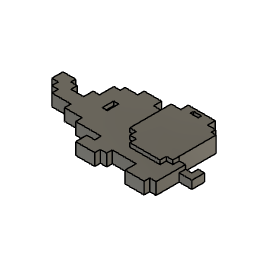
elephant pixel keychain v1 (Autodesk Fusion 360 design; units mm, degrees)
Autodesk Fusion 360 part; units mm, degrees
sketch "elephant sketch" plane through (0, 0, 0) normal (0, 0, 1) x (1, 0, 0)
  line L0 (5, 40) -> (5, 33)
  line L1 (5, 33) -> (9, 33)
  line L2 (9, 33) -> (9, 29)
  line L3 (9, 29) -> (13, 29)
  line L4 (13, 29) -> (13, 25)
  line L5 (13, 25) -> (25, 25)
  line L6 (25, 25) -> (25, 21)
  line L7 (25, 21) -> (36, 21)
  line L8 (36, 21) -> (36, 17)
  line L9 (36, 17) -> (52, 17)
  line L10 (52, 17) -> (52, 13)
  line L11 (52, 13) -> (47, 13)
  line L12 (47, 13) -> (47, 6)
  line L13 (47, 6) -> (59, 6)
  line L14 (59, 6) -> (59, 9.5)
  line L15 (59, 9.5) -> (63, 9.5)
  line L16 (63, 9.5) -> (63, 13)
  line L17 (63, 13) -> (78, 13)
  line L18 (78, 13) -> (78, 6)
  line L19 (78, 6) -> (90, 6)
  line L20 (90, 6) -> (90, 9.5)
  line L21 (90, 9.5) -> (94, 9.5)
  line L22 (94, 9.5) -> (94, 28)
  line L23 (94, 28) -> (90, 28)
  line L24 (90, 28) -> (90, 24)
  line L25 (90, 24) -> (86, 24)
  line L26 (86, 24) -> (86, 20)
  line L27 (86, 20) -> (67, 20)
  line L28 (67, 20) -> (67, 24)
  line L29 (67, 24) -> (63, 24)
  line L30 (63, 24) -> (63, 28)
  line L31 (63, 28) -> (59, 28)
  line L32 (59, 28) -> (59, 50)
  line L33 (59, 50) -> (52, 50)
  line L34 (52, 50) -> (52, 55)
  line L35 (52, 55) -> (41, 55)
  line L36 (41, 55) -> (41, 51)
  line L37 (41, 51) -> (33, 51)
  line L38 (33, 51) -> (33, 48)
  line L39 (33, 48) -> (29, 48)
  line L40 (29, 48) -> (29, 39)
  line L41 (29, 39) -> (25, 39)
  line L42 (25, 39) -> (25, 33)
  line L43 (25, 33) -> (17, 33)
  line L44 (17, 33) -> (17, 37)
  line L45 (17, 37) -> (13, 37)
  line L46 (13, 37) -> (13, 40)
  line L47 (13, 40) -> (5, 40)
  line L48 (94, 28) -> (98, 28)
  line L49 (98, 28) -> (98, 32)
  line L50 (98, 32) -> (102, 32)
  line L51 (102, 32) -> (102, 24)
  line L52 (102, 24) -> (94, 24)
  line L53 (59, 50) -> (59, 54)
  line L54 (59, 54) -> (65, 54)
  line L55 (65, 54) -> (65, 58.7382)
  line L56 (65, 58.7382) -> (81.9319, 58.7382)
  line L57 (81.9319, 58.7382) -> (81.9319, 54)
  line L58 (81.9319, 54) -> (87.0128, 54)
  line L59 (87.0128, 54) -> (87.0128, 51.2757)
  line L60 (87.0128, 51.2757) -> (90, 51.2757)
  line L61 (90, 51.2757) -> (90, 28)
  line L62 (36.8391, 40.0538) -> (36.8391, 32.8575)
  line L63 (36.8391, 32.8575) -> (40, 32.8575)
  line L64 (40, 32.8575) -> (40, 40.0538)
  line L65 (40, 40.0538) -> (36.8391, 40.0538)
  line L66 (71, 57) -> (75, 57)
  line L67 (75, 57) -> (75, 55)
  line L68 (75, 55) -> (70, 55)
  line L69 (70, 55) -> (70, 57)
  line L70 (70, 57) -> (71, 57)
  constraint vertical L0
  constraint perpendicular L0 L1
  constraint perpendicular L1 L2
  constraint perpendicular L0 L3
  constraint perpendicular L3 L4
  constraint perpendicular L0 L5
  constraint perpendicular L5 L6
  constraint perpendicular L6 L7
  constraint perpendicular L7 L8
  constraint perpendicular L8 L9
  constraint perpendicular L9 L10
  constraint perpendicular L10 L11
  constraint perpendicular L11 L12
  constraint perpendicular L12 L13
  constraint perpendicular L13 L14
  constraint perpendicular L14 L15
  constraint perpendicular L13 L16
  constraint perpendicular L16 L17
  constraint perpendicular L13 L18
  constraint perpendicular L18 L19
  constraint perpendicular L19 L20
  constraint perpendicular L20 L21
  constraint perpendicular L21 L22
  constraint perpendicular L22 L23
  constraint perpendicular L23 L24
  constraint perpendicular L22 L25
  constraint perpendicular L23 L26
  constraint perpendicular L22 L27
  constraint perpendicular L23 L28
  constraint perpendicular L28 L29
  constraint perpendicular L23 L30
  constraint perpendicular L30 L31
  constraint perpendicular L23 L32
  constraint perpendicular L30 L33
  constraint perpendicular L23 L34
  constraint perpendicular L34 L35
  constraint perpendicular L35 L36
  constraint perpendicular L34 L37
  constraint perpendicular L37 L38
  constraint perpendicular L38 L39
  constraint perpendicular L39 L40
  constraint perpendicular L38 L41
  constraint perpendicular L41 L42
  constraint perpendicular L42 L43
  constraint perpendicular L41 L44
  constraint perpendicular L44 L45
  constraint perpendicular L41 L46
  constraint perpendicular L0 L47
  constraint perpendicular L22 L48
  constraint perpendicular L23 L49
  constraint perpendicular L49 L50
  constraint perpendicular L50 L51
  constraint coincident L22 L52.end
  constraint perpendicular L22 L52
  constraint perpendicular L33 L53
  constraint perpendicular L32 L54
  constraint perpendicular L54 L55
  constraint perpendicular L55 L56
  constraint perpendicular L54 L57
  constraint perpendicular L57 L58
  constraint perpendicular L58 L59
  constraint perpendicular L59 L60
  constraint vertical L62
  constraint perpendicular L62 L63
  constraint perpendicular L63 L64
  constraint perpendicular L64 L65
  constraint parallel L56 L66
  constraint perpendicular L66 L67
  constraint perpendicular L67 L68
  constraint perpendicular L66 L69
  constraint perpendicular L69 L70
extrude "Extrude1" add sketch "elephant sketch" along normal blind 7.5 contours L0 L1 L2 L3 L4 L5 L6 L7 L8 L9 L10 L11 L12 L13 L14 L15 L16 L17 L18 L19 L20 L21 L22 L23 L24 L25 L26 L27 L28 L29 L30 L31 L32 L33 L34 L35 L36 L37 L38 L39 L40 L41 L42 L43 L44 L45 L46 L47
extrude "Extrude2" add sketch "elephant sketch" along normal blind 10 contours L24 L25 L26 L27 L28 L29 L30 L31 L32 L53 L54 L55 L56 L57 L58 L59 L60 L61 | L66 L67 L68 L69 L70
extrude "Extrude3" add sketch "elephant sketch" along normal blind 5 contours L22 L48 L49 L50 L51 L52
extrude "Extrude4" add sketch "elephant sketch" along normal blind 5 contours L62 L63 L64 L65
extrude "Extrude5" cut sketch "elephant sketch" along normal blind 13 contours L66 L67 L68 L69 L70
named bodies: "elephant keychain"
